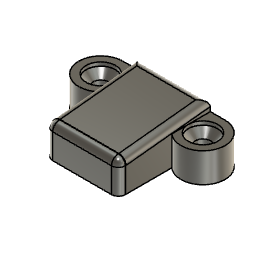
fishing (Autodesk Fusion 360 design; units mm, degrees)
Autodesk Fusion 360 part; units mm, degrees
sketch "Sketch1" plane through (0, 0, 0) normal (0, 0, 1) x (1, 0, 0)
  line L0 (0, 0) -> (19.8, 0)
  line L1 (19.8, 0) -> (19.8, 25)
  line L2 (19.8, 25) -> (0, 25)
  line L3 (0, 25) -> (0, 0)
  dimension "d1" = 19.8
  dimension "d2" = 25
  constraint horizontal L0
  constraint vertical L1
  constraint horizontal L2
  constraint vertical L3
  constraint coincident L0.start L3.end
  measures "d1" distance of L0.start L0.end
  measures "d2" distance of L0.start L2.end
extrude "Extrude1" add sketch "Sketch1" along normal blind 2
sketch "Sketch2" plane through (19.8, 0, 0) normal (1, 0, 0) x (0, 1, 0)
  line L0 (0, 0) -> (25, 0)
  line L1 (25, 0) -> (25, 2)
  line L2 (25, 2) -> (0, 2)
  line L3 (0, 2) -> (0, 0)
  line L4 (0, 2) -> (0, 8.7)
  line L5 (0, 8.7) -> (2, 8.7)
  line L6 (25, 2) -> (25, 11.1)
  line L7 (2, 8.7) -> (25, 11.1)
  dimension "d5" = 9.1
  dimension "d6" = 6.7
  constraint coincident L2.end L3.start
  constraint perpendicular L2 L4
  constraint perpendicular L4 L5
  constraint coincident L1.end L2.start
  constraint perpendicular L2 L6
  measures "d5" distance of L1.end L6.end
  measures "d6" distance of L2.end L4.end
extrude "Extrude2" add sketch "Sketch2" against normal blind 19.8 contours L2 L4 L5 L6 L7
shell "Shell1" thickness 2 removed faces 1 at (13.2, 25, 3.7)
sketch "Sketch4" plane through (0, 0, 0) normal (0, 0, -1) x (1, 0, 0)
  line L0 (0, 0) -> (0, -25)
  line L1 (0, -25) -> (19.8, -25)
  line L2 (19.8, -25) -> (19.8, 0)
  line L3 (19.8, 0) -> (0, 0)
  circle A0 centre (23.8, -19) radius 6
  line L4 (17.8, -19) -> (17.8, -25)
  line L5 (17.8, -25) -> (23.8, -25)
  circle A1 centre (-4, -19) radius 6
  line L6 (2, -19) -> (2, -25)
  line L7 (-4, -25) -> (2, -25)
  dimension "d30" = 15.8
  constraint coincident A0 L4.start
  constraint coincident L1 L4.end
  constraint tangent A0 L4
  constraint perpendicular L1 L4
  constraint coincident A0 L5.end
  constraint tangent A0 L5
  constraint perpendicular L4 L5
  constraint coincident A1 L6.start
  constraint coincident L1 L6.end
  constraint tangent A1 L6
  constraint perpendicular L1 L6
  constraint coincident A1 L7.start
  constraint tangent A1 L7
  measures "d30" distance of L4.end L6.end
extrude "Extrude3" add sketch "Sketch4" against normal blind 8 contours L0 A1 | L0 A1 L7 | L2 A0 | L2 A0 L5 picked at (-3.5605, -18.3377) picked at (24.5296, -17.6528)
sketch "Sketch5" plane through (0, 0, 8) normal (0, 0, 1) x (-1, 0, 0)
  arc A0 (4, -25) -> (0, -14.5279) centre (4, -19) ccw
  line L0 (0, -14.5279) -> (0, -25)
  line L1 (0, -25) -> (4, -25)
  circle A1 centre (4, -19) radius 4
  circle A2 centre (-23.8, -19) radius 4
  dimension "d31" = 27.8
  constraint concentric A0 A1
  constraint tangent L0 A1
  measures "d31" distance of A0.centre A2.centre
extrude "Extrude4" cut sketch "Sketch5" against normal blind 1 contours A1 | A2
sketch "Sketch6" plane through (0, 0, 7) normal (0, 0, 1) x (-1, 0, 0)
  circle A0 centre (4, -19) radius 4
  circle A1 centre (4, -19) radius 2.075
  circle A2 centre (-23.8, -19) radius 2.075
  dimension "d18" = 4.15
  dimension "d19" = 4.15
  dimension "d32" = 27.8
  constraint concentric A0 A1
  measures "d18" diameter of A1
  measures "d19" diameter of A2
  measures "d32" distance of A0.centre A2.centre
extrude "Extrude5" cut sketch "Sketch6" against normal blind 17 contours A1 | A2
chamfer "Chamfer1" distance 1.9 angle 45 2 edges at (-2.0654, 18.2496, 7) (25.7346, 18.2496, 7)
fillet "Fillet1" radius 1.9 8 edges at (9.9, 0, 8.7) (0, 13.5, 9.9) (0, 1, 8.7) (19.8, 13.5, 9.9) (9.9, 25, 11.1) (19.8, 1, 8.7) (19.8, 0, 4.35) (0, 0, 4.35)
fillet "Fillet2" [suppressed]
equation "d1 = Width + 2 mm + 2 mm"
equation "d5 = DepthHigh + 2 mm"
equation "d6 = DepthLow + 2 mm"
equation "d7 = -Width - 2 mm - 2 mm"
equation "Width = 15.8 mm" comment "Normal: 15"
equation "DepthLow = 4.7 mm" comment "Lille:4,0 Stor 4,7"
equation "DepthHigh = 7.1 mm" comment "Lille:6,4 Stor:7,1"
equation "d30 = Width"
equation "d31 = Width + 12 mm"
equation "d32 = Width + 12 mm"
